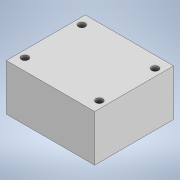
# Autodesk Inventor part: Box
Saved by Autodesk Inventor 2022 (Build 260153000, 153)
## iProperties
Created: 2023-02-07
Part Number: Box
Material: Generic
Document SubType Name: Modeling
Designer: Deven Joshi
Density: 1 g/cm^3
Appearance: Default
Author: Deven Joshi
Autodesk Inventor part; units mm, degrees
ref_plane "YZ Plane" through (0, 0, 0) normal (1, 0, 0) x (0, 1, 0)
ref_plane "XZ Plane" through (0, 0, 0) normal (0, 1, 0) x (-1, 0, 0)
ref_plane "XY Plane" through (0, 0, 0) normal (0, 0, 1) x (1, 0, 0)
sketch "Sketch1" plane through (0, 0, 0) normal (0, 1, 0) x (-1, 0, 0)
  line L0 (-19, -17) -> (19, -17)
  line L1 (19, -17) -> (19, 17)
  line L2 (19, 17) -> (-19, 17)
  line L3 (-19, 17) -> (-19, -17)
  line L4 (-19, -17) -> (19, 17) construction
  line L5 (19, -17) -> (-19, 17) construction
  point P0 (0, 0)
  dimension "d0" = 38
  dimension "d1" = 34
  constraints: 12 end point, 2 midpoint, 2 parallel, 1 horizontal, 1 perpendicular
  measures "d0" distance of L2.end L1.end
  measures "d1" distance of L1.end L0.end
extrude "Extrusion1" add sketch "Sketch1" along normal blind 20
sketch "Sketch2" plane through (0, 0, 0) normal (0, -1, 0) x (1, 0, 0)
  arc A0 (0, 10) -> (0, -10) centre (0, 0) ccw
  line L0 (0, 10) -> (0, -23.7919) construction
  line L1 (0, -10) -> (0, 10)
  dimension "d4" = 20
  constraints: 4 end point, 2 point on circle, 2 point on line, 1 centre point, 1 coincident, 1 collinear, 1 vertical
  measures "d4" diameter of A0
revolve "Revolution1" cut sketch "Sketch2" angle 180 about axis through (0, 0, 10) along (0, 0, -1)
sketch "Sketch3" plane through (0, 0, 0) normal (0, -1, 0) x (1, 0, 0)
  point P0 (0, 0)
  point P1 (16, 12)
  point P2 (16, -12)
  point P3 (-16, -12.4929)
  point P4 (-16, 12)
hole "Hole1" at (-16, 0, -12.4929) at (-16, 0, 12) at (16, 0, 12) at (16, 0, -12) direction (0, 1, 0) diameter 3 end through all
body "Solid1"
